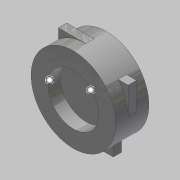
# Autodesk Inventor part: CHECK VALVE DISK WAFER 316L DN40
Saved by Autodesk Inventor 2017 (Build 210142000, 142)
## iProperties
Created: 2015-03-19
Part Number: CHECK VALVE DISK WAFER 316L DN40
Material: 304L
Document SubType Name: Modeling
Designer: m_crauwels
Density: 8 g/cm^3
Appearance: Steel
Mass: 365.342 g
Surface Area: 480.363 cm^2
Volume: 45.6678 cm^3
Description: BV38-6666E-PN10/PN16
Catalog Web Link: http://www.pocketbrewery.com
PipeDiameter: 48.000 mm
DiamExt: 80.000 mm
Thickness: 31.500 mm
Author: m_crauwels
Autodesk Inventor part; units mm, degrees
ref_plane "YZ Plane" through (0, 0, 0) normal (1, 0, 0) x (0, 1, 0)
ref_plane "XZ Plane" through (0, 0, 0) normal (0, 1, 0) x (-1, 0, 0)
ref_plane "XY Plane" through (0, 0, 0) normal (0, 0, 1) x (1, 0, 0)
sketch "Sketch1" plane through (0, 0, 0) normal (0, 1, 0) x (-1, 0, 0)
  line L0 (15.75, 0) -> (-15.75, 0) construction
  line L1 (15.75, 40) -> (-15.75, 40)
  line L2 (-15.75, 40) -> (-15.75, 24)
  line L3 (15.75, 24) -> (-15.75, 24)
  line L4 (15.75, 24) -> (15.75, 40)
  line L5 (3.9375, 0) -> (-3.9375, 0)
  line L6 (-3.9375, 0) -> (-3.9375, 24)
  line L7 (-3.9375, 24) -> (3.9375, 24)
  line L8 (3.9375, 24) -> (3.9375, 0)
  line L9 (3.9375, 0) -> (-3.9375, 24) construction
  line L10 (-3.9375, 0) -> (3.9375, 24) construction
  point P0 (0, 12)
  point P1 (0, 24)
  point P2 (0, 0)
  point P3 (0, 0)
  dimension "Thickness" = 31.5
  dimension "DiamExt" = 80
  dimension "PipeDiameter" = 48
  dimension "d8" = 7.875
  constraints: 22 end point, 6 midpoint, 4 perpendicular, 2 horizontal, 2 parallel, 1 coincident, 1 point on line
  measures "Thickness" distance of L1.start L1.end
  measures "DiamExt" diameter of L1 L0
  measures "PipeDiameter" diameter of L3 L0
  measures "d8" distance of L6.end L7.end
revolve "Revolution1" add sketch "Sketch1" angle 360 about axis through (-15.75, 0, 0) along (1, 0, 0)
sketch "Sketch5" plane through (-3.9375, 0, 0) normal (-1, 0, 0) x (0, 0, 1)
  circle A0 centre (0, 0) radius 40 projected
  line L0 (0, 0) -> (33.9411, 33.9411) construction
  line L1 (0, 0) -> (48, 0) construction
  circle A1 centre (33.9411, 33.9411) radius 8 construction
  circle A2 centre (0, 0) radius 40 projected
  line L2 (40, 0) -> (40, 25.9411)
  line L3 (40, 25.9411) -> (30.4476, 25.9411)
  point P0 (0, 0)
  dimension "d18" = 45
  dimension "d19" = 16
  constraints: 8 end point, 2 perpendicular, 2 point on circle, 2 tangent, 1 centre point, 1 equal length, 1 horizontal, 1 point on line, 1 vertical, 3 other
  measures "d18" angle of L1 L0
  measures "d19" diameter of A1
extrude "Extrusion1" add sketch "Sketch5" against normal up to surface (7.875 mm away) from surface at 0 contours A0 L3 L2
pattern_circular "Circular Pattern1" count 4 over 360 about axis through (0, 0, 0) along (-1, 0, 0) of "Extrusion1"
equation "\"d8\" = 0.25 * Thickness"
body "Solid1"
